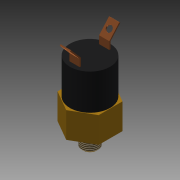
# Autodesk Inventor part: fc16-069
Saved by Autodesk Inventor 2016 SP1 (Build 200210100, 210)
## iProperties
Category: Electronics
Company: Autodesk, Inc.
Shininess: 64.0
Length Units: 11272
Angle Units: 11279
Time Units: 11290
Mass Units: 11283
Length Display Precision: 3
Angle Display Precision: 2
Compacted: True
Part Number: fc16-069
Document SubType Name: Modeling
Created: 2015-11-24
Manufacturer: Standard
Standards Organization: Custom
Catalog Web Link: http://files.andymark.com/NasonSMspecs.pdf
Description: Pressure Switch
Vendor: NASON
Density: 1 g/cm^3
Material: Generic
Designer: Autodesk, Inc.
Appearance: Default
Density: 0.0
Volumn: 0.0
Area: 0.0
PropertySet Name: Model Information
Control State: 0
Master: False
Checked Out: False
Title: Pressure Switch
Author: Autodesk, Inc.
Keywords: FIRSTChoice
Autodesk Inventor part; units mm, degrees
ref_plane "YZ Plane" through (0, 0, 0) normal (1, 0, 0) x (0, 1, 0)
ref_plane "XZ Plane" through (0, 0, 0) normal (0, 1, 0) x (-1, 0, 0)
ref_plane "XY Plane" through (0, 0, 0) normal (0, 0, 1) x (1, 0, 0)
sketch "Sketch1" plane through (0, 0, 0) normal (0, 0, 1) x (1, 0, 0)
  line L0 (0, 14.6647) -> (12.7, 7.3323)
  line L1 (12.7, 7.3323) -> (12.7, -7.3323)
  line L2 (12.7, -7.3323) -> (0, -14.6647)
  line L3 (0, -14.6647) -> (-12.7, -7.3323)
  line L4 (-12.7, -7.3323) -> (-12.7, 7.3323)
  line L5 (-12.7, 7.3323) -> (0, 14.6647)
  line L6 (0, 14.6647) -> (0, 0)
  dimension "d0" = 25.4
  constraints: 14 end point, 1 coincident, 1 parallel, 1 vertical, 11 other
  measures "d0" distance between parallel lines of L2 L5
extrude "Extrusion1" add sketch "Sketch1" along normal blind 15.875
sketch "Sketch2" plane through (0, 0, 0) normal (0, 0, -1) x (-1, 0, 0)
  line L0 (12.7, -7.3323) -> (12.7, 7.3323) projected
  line L1 (12.7, 7.3323) -> (0, 14.6647) projected
  line L2 (0, 14.6647) -> (-12.7, 7.3323) projected
  line L3 (-12.7, 7.3323) -> (-12.7, -7.3323) projected
  line L4 (-12.7, -7.3323) -> (0, -14.6647) projected
  line L5 (0, -14.6647) -> (12.7, -7.3323) projected
  line L6 (-6.35, 10.9985) -> (6.35, -10.9985) construction
  circle A0 centre (0, 0) radius 5.08
  dimension "d3" = 10.16
  constraints: 3 midpoint, 2 end point, 1 centre point
  measures "d3" diameter of A0
extrude "Extrusion2" add sketch "Sketch2" along normal blind 11.049 contours A0
sketch "Sketch3" plane through (0, 0, -11.049) normal (0, 0, -1) x (-1, 0, 0)
  circle A0 centre (0, 0) radius 5.08 projected
  circle A1 centre (0, 0) radius 1.5875
  dimension "d6" = 3.175
  constraints: 1 centre point, 1 coincident
  measures "d6" diameter of A1
extrude "Extrusion3" cut sketch "Sketch3" against normal blind 19.9898 contours A1
sketch "Sketch4" plane through (0, 0, 15.875) normal (0, 0, 1) x (1, 0, 0)
  line L0 (12.7, 7.3323) -> (12.7, -7.3323) projected
  line L1 (0, 14.6647) -> (12.7, 7.3323) projected
  line L2 (-12.7, 7.3323) -> (0, 14.6647) projected
  line L3 (-12.7, -7.3323) -> (-12.7, 7.3323) projected
  line L4 (0, -14.6647) -> (-12.7, -7.3323) projected
  line L5 (12.7, -7.3323) -> (0, -14.6647) projected
  line L6 (-6.35, 10.9985) -> (6.35, -10.9985)
  circle A0 centre (0, 0) radius 12.3825
  dimension "d9" = 24.765
  constraints: 4 midpoint, 2 end point, 1 centre point
  measures "d9" diameter of A0
extrude "Extrusion4" add sketch "Sketch4" along normal blind 21.971 contours A0 L6 | L6 A0
sketch "Sketch5" plane through (0, 0, 0) normal (1, 0, 0) x (0, 1, 0)
  line L0 (12.3825, 15.875) -> (12.3825, 37.846) projected
  line L1 (-12.3825, 37.846) -> (12.3825, 37.846) projected
  line L2 (-12.3825, 15.875) -> (12.3825, 15.875) projected
  line L3 (9.525, 37.846) -> (9.525, 42.2598)
  line L4 (9.525, 42.2598) -> (15.5086, 49.1328)
  line L5 (15.5086, 49.1328) -> (14.9339, 49.6332)
  line L6 (14.9339, 49.6332) -> (8.763, 42.545)
  line L7 (8.763, 42.545) -> (8.763, 37.846)
  line L8 (0, 37.846) -> (0, 32.3818)
  line L9 (-12.3825, 15.875) -> (-12.3825, 37.846)
  line L10 (12.3825, 37.846) -> (-12.3825, 37.846)
  line L11 (-9.525, 37.846) -> (-9.525, 42.2598)
  line L12 (-9.525, 42.2598) -> (-15.5086, 49.1328)
  line L13 (-15.5086, 49.1328) -> (-14.9339, 49.6332)
  line L14 (-14.9339, 49.6332) -> (-8.763, 42.545)
  line L15 (-8.763, 42.545) -> (-8.763, 37.846)
  dimension "d12" = 19.05
  dimension "d13" = 0.762
  dimension "d14" = 0.762
  dimension "d15" = 4.699
  dimension "d17" = 9.398
  constraints: 26 end point, 10 symmetric about line, 4 perpendicular, 4 point on line, 1 midpoint, 1 parallel, 7 other
  measures "d12" distance between parallel lines of L11 L3
  measures "d13" distance between parallel lines of L7 L3
  measures "d14" distance between parallel lines of L6 L4
  measures "d15" distance of L6.end L7.end
  measures "d17" distance of L5.end L6.end
extrude "Extrusion5" add sketch "Sketch5" along normal mid plane 6.35 contours L1 L7 L6 L5 L4 L3 | L11 L12 L13 L14 L15 L1
sketch "Sketch6" plane through (-3.175, -8.763, 42.545) normal (0, 0.7542, 0.6566) x (1, 0, 0)
  line L0 (6.35, -9.398) -> (6.35, 0) projected
  line L1 (0, 0) -> (6.35, 0) projected
  line L2 (0, 0) -> (0, -9.398) projected
  line L3 (0, -9.398) -> (6.35, -9.398) projected
  circle A0 centre (3.175, -4.699) radius 1.8713
  constraints: 1 centre point
extrude "Extrusion6" cut sketch "Sketch6" against normal blind 6.35 contours A0
mirror "Mirror1" about plane through (0, 0, 0) normal (0, 1, 0) of "Extrusion6"
thread "Thread1" size "1/8" designation "1/8 - 27 NPT" standard "NPT" full length
chamfer "Chamfer1" distance 1 angle 45 1 edges at (5.08, 0, -11.049)
fillet "Fillet1" radius 3.175 1 edges at (5.08, 0, 0)
equation "\"d14\" = d13"
body "Solid1"
